Autodesk Fusion 360 part; units mm, degrees
(part 8 of 20)
  spline S469 degree 3 poles (28.0099, -86.4526) (27.9329, -86.3989) (27.7756, -86.2891) (27.5841, -86.2754) (27.4864, -86.2684) knots 0 0 0 0 0.027619 0.056426 0.056426 0.056426 0.056426
  spline S470 degree 3 poles (27.4864, -86.2684) (27.3397, -86.2815) (27.0506, -86.3072) (26.8376, -86.504) (26.7326, -86.6009) knots 0 0 0 0 0.04285 0.084486 0.084486 0.084486 0.084486
  spline S471 degree 3 poles (26.7326, -86.6009) (26.6484, -86.7405) (26.4545, -87.062) (26.447, -87.4395) (26.4427, -87.6531) knots 0 0 0 0 0.048123 0.11083 0.11083 0.11083 0.11083
  spline S472 degree 3 poles (26.4427, -87.6531) (26.4463, -87.8689) (26.4526, -88.2476) (26.6412, -88.5736) (26.7224, -88.7138) knots 0 0 0 0 0.063398 0.111295 0.111295 0.111295 0.111295
  spline S473 degree 3 poles (26.7224, -88.7138) (26.8235, -88.8103) (27.0281, -89.0055) (27.3098, -89.0315) (27.4523, -89.0447) knots 0 0 0 0 0.040675 0.082263 0.082263 0.082263 0.082263
  spline S474 degree 3 poles (27.4523, -89.0447) (27.5666, -89.0365) (27.7895, -89.0205) (27.9687, -88.8876) (28.0559, -88.823) knots 0 0 0 0 0.033628 0.065508 0.065508 0.065508 0.065508
  spline S475 degree 3 poles (28.0559, -88.823) (28.13, -88.733) (28.2935, -88.5344) (28.3383, -88.28) (28.3629, -88.1409) knots 0 0 0 0 0.034396 0.07593 0.07593 0.07593 0.07593
  spline S476 degree 3 poles (21.9679, -37.0341) (21.9715, -36.7658) (21.9781, -36.2826) (22.0973, -35.8148) (22.1504, -35.6068) knots 0 0 0 0 0.080152 0.144341 0.144341 0.144341 0.144341
  spline S477 degree 3 poles (22.1504, -35.6068) (22.215, -35.4399) (22.3376, -35.1234) (22.5787, -34.8854) (22.6927, -34.7729) knots 0 0 0 0 0.052977 0.10048 0.10048 0.10048 0.10048
  spline S478 degree 3 poles (22.6927, -34.7729) (22.8241, -34.6874) (23.0989, -34.5085) (23.427, -34.4895) (23.5982, -34.4795) knots 0 0 0 0 0.046203 0.096661 0.096661 0.096661 0.096661
  spline S479 degree 3 poles (23.5982, -34.4795) (23.726, -34.4851) (23.9715, -34.4958) (24.1964, -34.5943) (24.3042, -34.6415) knots 0 0 0 0 0.037989 0.072993 0.072993 0.072993 0.072993
  spline S480 degree 3 poles (24.3042, -34.6415) (24.4015, -34.7022) (24.5988, -34.8254) (24.736, -35.0134) (24.8056, -35.1088) knots 0 0 0 0 0.034048 0.069103 0.069103 0.069103 0.069103
  spline S481 degree 3 poles (24.8056, -35.1088) (24.8689, -35.2198) (25.0029, -35.4547) (25.0769, -35.715) (25.116, -35.8523) knots 0 0 0 0 0.038176 0.080832 0.080832 0.080832 0.080832
  spline S482 degree 3 poles (25.116, -35.8523) (25.1487, -36.0234) (25.2232, -36.4135) (25.2266, -36.8109) (25.2285, -37.0341) knots 0 0 0 0 0.052146 0.118926 0.118926 0.118926 0.118926
  spline S483 degree 3 poles (25.2285, -37.0341) (25.2249, -37.3007) (25.2183, -37.7815) (25.1003, -38.2472) (25.0477, -38.4546) knots 0 0 0 0 0.079639 0.143634 0.143634 0.143634 0.143634
  spline S484 degree 3 poles (25.0477, -38.4546) (24.9836, -38.6216) (24.8617, -38.9385) (24.621, -39.1773) (24.5072, -39.2903) knots 0 0 0 0 0.052961 0.100531 0.100531 0.100531 0.100531
  spline S485 degree 3 poles (24.5072, -39.2903) (24.3755, -39.3763) (24.0998, -39.5564) (23.7704, -39.5754) (23.5982, -39.5853) knots 0 0 0 0 0.046338 0.097057 0.097057 0.097057 0.097057
  spline S486 degree 3 poles (23.5982, -39.5853) (23.372, -39.566) (22.9307, -39.5283) (22.6159, -39.218) (22.4625, -39.0669) knots 0 0 0 0 0.065835 0.128409 0.128409 0.128409 0.128409
  spline S487 degree 3 poles (22.4625, -39.0669) (22.319, -38.7988) (21.9814, -38.1677) (21.9729, -37.448) (21.9679, -37.0341) knots 0 0 0 0 0.090022 0.211899 0.211899 0.211899 0.211899
  line L97 (28.3868, -38.1733) -> (28.9904, -38.2517)
  spline S488 degree 3 poles (28.9904, -38.2517) (28.9478, -38.4456) (28.866, -38.8173) (28.6076, -39.0957) (28.484, -39.2289) knots 0 0 0 0 0.058356 0.111856 0.111856 0.111856 0.111856
  spline S489 degree 3 poles (28.484, -39.2289) (28.3379, -39.3318) (28.0378, -39.5433) (27.6711, -39.5688) (27.4829, -39.5819) knots 0 0 0 0 0.052559 0.107965 0.107965 0.107965 0.107965
  spline S490 degree 3 poles (27.4829, -39.5819) (27.2499, -39.5644) (26.7983, -39.5304) (26.4541, -39.2376) (26.2875, -39.0958) knots 0 0 0 0 0.068154 0.132052 0.132052 0.132052 0.132052
  spline S491 degree 3 poles (26.2875, -39.0958) (26.156, -38.9051) (25.8681, -38.4877) (25.847, -37.9789) (25.8356, -37.7026) knots 0 0 0 0 0.068157 0.149141 0.149141 0.149141 0.149141
  spline S492 degree 3 poles (25.8356, -37.7026) (25.8419, -37.5174) (25.8539, -37.1649) (25.9733, -36.8333) (26.03, -36.676) knots 0 0 0 0 0.055211 0.105055 0.105055 0.105055 0.105055
  spline S493 degree 3 poles (26.03, -36.676) (26.1022, -36.5391) (26.2444, -36.2695) (26.4973, -36.0996) (26.6218, -36.016) knots 0 0 0 0 0.04564 0.089884 0.089884 0.089884 0.089884
  spline S494 degree 3 poles (26.6218, -36.016) (26.7577, -35.9519) (27.0316, -35.8226) (27.334, -35.8049) (27.4863, -35.7961) knots 0 0 0 0 0.044643 0.089955 0.089955 0.089955 0.089955
  spline S495 degree 3 poles (27.4863, -35.7961) (27.6701, -35.8054) (28.018, -35.8232) (28.3126, -36.0075) (28.4516, -36.0945) knots 0 0 0 0 0.054149 0.102527 0.102527 0.102527 0.102527
  spline S496 degree 3 poles (28.4516, -36.0945) (28.566, -36.208) (28.8051, -36.445) (28.8888, -36.7718) (28.9325, -36.942) knots 0 0 0 0 0.047449 0.099081 0.099081 0.099081 0.099081
  line L98 (28.9325, -36.942) -> (28.3356, -37.0341)
  spline S497 degree 3 poles (28.3356, -37.0341) (28.3047, -36.9227) (28.2473, -36.7153) (28.1013, -36.5579) (28.0338, -36.485) knots 0 0 0 0 0.034086 0.063475 0.063475 0.063475 0.063475
  spline S498 degree 3 poles (28.0338, -36.485) (27.9568, -36.4313) (27.7995, -36.3216) (27.608, -36.3078) (27.5102, -36.3008) knots 0 0 0 0 0.027619 0.056426 0.056426 0.056426 0.056426
  spline S499 degree 3 poles (27.5102, -36.3008) (27.3636, -36.3139) (27.0744, -36.3396) (26.8614, -36.5364) (26.7565, -36.6334) knots 0 0 0 0 0.04285 0.084486 0.084486 0.084486 0.084486
  spline S500 degree 3 poles (26.7565, -36.6334) (26.6723, -36.7729) (26.4784, -37.0944) (26.4708, -37.4719) (26.4666, -37.6855) knots 0 0 0 0 0.048123 0.11083 0.11083 0.11083 0.11083
  spline S501 degree 3 poles (26.4666, -37.6855) (26.4702, -37.9013) (26.4764, -38.28) (26.6651, -38.606) (26.7462, -38.7463) knots 0 0 0 0 0.063398 0.111295 0.111295 0.111295 0.111295
  spline S502 degree 3 poles (26.7462, -38.7463) (26.8474, -38.8427) (27.0519, -39.0379) (27.3337, -39.0639) (27.4761, -39.0771) knots 0 0 0 0 0.040675 0.082263 0.082263 0.082263 0.082263
  spline S503 degree 3 poles (27.4761, -39.0771) (27.5905, -39.0689) (27.8133, -39.0529) (27.9926, -38.92) (28.0798, -38.8554) knots 0 0 0 0 0.033628 0.065508 0.065508 0.065508 0.065508
  spline S504 degree 3 poles (28.0798, -38.8554) (28.1538, -38.7654) (28.3173, -38.5668) (28.3622, -38.3124) (28.3868, -38.1733) knots 0 0 0 0 0.034395 0.07593 0.07593 0.07593 0.07593
  line L99 (29.5157, -39.5) -> (29.5157, -35.8779)
  line L100 (29.5157, -35.8779) -> (30.0648, -35.8779)
  line L101 (30.0648, -35.8779) -> (30.0648, -36.3861)
  spline S505 degree 3 poles (30.0648, -36.3861) (30.1267, -36.3015) (30.2516, -36.131) (30.429, -36.016) (30.5184, -35.9581) knots 0 0 0 0 0.031158 0.062835 0.062835 0.062835 0.062835
  spline S506 degree 3 poles (30.5184, -35.9581) (30.6176, -35.9108) (30.8215, -35.8137) (31.0471, -35.802) (31.163, -35.7961) knots 0 0 0 0 0.032617 0.067048 0.067048 0.067048 0.067048
  spline S507 degree 3 poles (31.163, -35.7961) (31.2875, -35.8008) (31.5199, -35.8096) (31.7269, -35.9145) (31.823, -35.9632) knots 0 0 0 0 0.036859 0.068796 0.068796 0.068796 0.068796
  spline S508 degree 3 poles (31.823, -35.9632) (31.9027, -36.0249) (32.0636, -36.1496) (32.1451, -36.3362) (32.1862, -36.4304) knots 0 0 0 0 0.029725 0.060035 0.060035 0.060035 0.060035
  spline S509 degree 3 poles (32.1862, -36.4304) (32.3364, -36.2455) (32.6275, -35.8869) (33.0839, -35.8257) (33.3049, -35.7961) knots 0 0 0 0 0.068625 0.133023 0.133023 0.133023 0.133023
  spline S510 degree 3 poles (33.3049, -35.7961) (33.47, -35.8045) (33.7779, -35.8202) (34.021, -36.0076) (34.1337, -36.0945) knots 0 0 0 0 0.048244 0.08997 0.08997 0.08997 0.08997
  spline S511 degree 3 poles (34.1337, -36.0945) (34.218, -36.2168) (34.4074, -36.4917) (34.4178, -36.8274) (34.4236, -37.0137) knots 0 0 0 0 0.043695 0.098195 0.098195 0.098195 0.098195
  line L102 (34.4236, -37.0137) -> (34.4236, -39.5)
  line L103 (34.4236, -39.5) -> (33.8131, -39.5)
  line L104 (33.8131, -39.5) -> (33.8131, -37.2183)
  spline S512 degree 3 poles (33.8131, -37.2183) (33.8131, -37.1121) (33.813, -36.9328) (33.7707, -36.7588) (33.7534, -36.6879) knots 0 0 0 0 0.031711 0.053535 0.053535 0.053535 0.053535
  spline S513 degree 3 poles (33.7534, -36.6879) (33.729, -36.6363) (33.6791, -36.5309) (33.5849, -36.4621) (33.5368, -36.427) knots 0 0 0 0 0.016863 0.034394 0.034394 0.034394 0.034394
  spline S514 degree 3 poles (33.5368, -36.427) (33.4811, -36.3982) (33.3657, -36.3384) (33.2357, -36.3316) (33.1685, -36.3281) knots 0 0 0 0 0.018597 0.038532 0.038532 0.038532 0.038532
  spline S515 degree 3 poles (33.1685, -36.3281) (33.0473, -36.3379) (32.8094, -36.3572) (32.6247, -36.5081) (32.5341, -36.5822) knots 0 0 0 0 0.035532 0.069798 0.069798 0.069798 0.069798
  spline S516 degree 3 poles (32.5341, -36.5822) (32.4608, -36.6889) (32.2936, -36.9321) (32.286, -37.229) (32.2817, -37.3956) knots 0 0 0 0 0.038079 0.086792 0.086792 0.086792 0.086792
  line L105 (32.2817, -37.3956) -> (32.2817, -39.5)
  line L106 (32.2817, -39.5) -> (31.6678, -39.5)
  line L107 (31.6678, -39.5) -> (31.6678, -37.1467)
  spline S517 degree 3 poles (31.6678, -37.1467) (31.6654, -37.0246) (31.6611, -36.8078) (31.5613, -36.6164) (31.5177, -36.5328) knots 0 0 0 0 0.036008 0.063954 0.063954 0.063954 0.063954
  spline S518 degree 3 poles (31.5177, -36.5328) (31.4555, -36.4732) (31.3193, -36.3428) (31.1296, -36.3333) (31.0266, -36.3281) knots 0 0 0 0 0.025037 0.054812 0.054812 0.054812 0.054812
  spline S519 degree 3 poles (31.0266, -36.3281) (30.9418, -36.3338) (30.7724, -36.3451) (30.6224, -36.4248) (30.5474, -36.4645) knots 0 0 0 0 0.025172 0.050327 0.050327 0.050327 0.050327
  spline S520 degree 3 poles (30.5474, -36.4645) (30.4788, -36.5162) (30.3385, -36.6218) (30.2657, -36.7818) (30.2285, -36.8636) knots 0 0 0 0 0.025339 0.051812 0.051812 0.051812 0.051812
  spline S521 degree 3 poles (30.2285, -36.8636) (30.1998, -36.9699) (30.133, -37.2174) (30.1308, -37.4742) (30.1296, -37.6207) knots 0 0 0 0 0.032907 0.076633 0.076633 0.076633 0.076633
  line L108 (30.1296, -37.6207) -> (30.1296, -39.5)
  line L109 (30.1296, -39.5) -> (29.5157, -39.5)
  spline S522 degree 3 poles (19.028, -36.7885) (18.9112, -36.7401) (18.6922, -36.6493) (18.5352, -36.4722) (18.4618, -36.3895) knots 0 0 0 0 0.037333 0.070073 0.070073 0.070073 0.070073
  spline S523 degree 3 poles (18.4618, -36.3895) (18.4081, -36.2969) (18.2969, -36.1051) (18.2842, -35.8834) (18.2776, -35.7688) knots 0 0 0 0 0.031652 0.065561 0.065561 0.065561 0.065561
  spline S524 degree 3 poles (18.2776, -35.7688) (18.2938, -35.5943) (18.326, -35.2463) (18.5554, -34.9827) (18.6698, -34.8513) knots 0 0 0 0 0.05117 0.102058 0.102058 0.102058 0.102058
  spline S525 degree 3 poles (18.6698, -34.8513) (18.8165, -34.7429) (19.1259, -34.5144) (19.511, -34.4915) (19.7135, -34.4795) knots 0 0 0 0 0.053536 0.112931 0.112931 0.112931 0.112931
  spline S526 degree 3 poles (19.7135, -34.4795) (19.9176, -34.4921) (20.307, -34.5161) (20.6189, -34.749) (20.7674, -34.8598) knots 0 0 0 0 0.059849 0.114229 0.114229 0.114229 0.114229
  spline S527 degree 3 poles (20.7674, -34.8598) (20.8838, -34.9932) (21.1159, -35.2592) (21.1496, -35.6106) (21.1664, -35.7858) knots 0 0 0 0 0.051706 0.103118 0.103118 0.103118 0.103118
  spline S528 degree 3 poles (21.1664, -35.7858) (21.1597, -35.8968) (21.1464, -36.1132) (21.0372, -36.3002) (20.984, -36.3912) knots 0 0 0 0 0.032847 0.064022 0.064022 0.064022 0.064022
  spline S529 degree 3 poles (20.984, -36.3912) (20.9118, -36.4734) (20.7582, -36.6484) (20.5436, -36.74) (20.4297, -36.7885) knots 0 0 0 0 0.032377 0.06897 0.06897 0.06897 0.06897
  spline S530 degree 3 poles (20.4297, -36.7885) (20.5721, -36.8436) (20.8449, -36.9492) (21.0382, -37.1681) (21.1306, -37.2729) knots 0 0 0 0 0.045038 0.086311 0.086311 0.086311 0.086311
  spline S531 degree 3 poles (21.1306, -37.2729) (21.2007, -37.392) (21.3456, -37.6382) (21.3624, -37.9236) (21.3711, -38.0709) knots 0 0 0 0 0.040859 0.084421 0.084421 0.084421 0.084421
  spline S532 degree 3 poles (21.3711, -38.0709) (21.3526, -38.2758) (21.3157, -38.6833) (21.0498, -38.9941) (20.9175, -39.1487) knots 0 0 0 0 0.060084 0.11955 0.11955 0.11955 0.11955
  spline S533 degree 3 poles (20.9175, -39.1487) (20.7492, -39.276) (20.3968, -39.5425) (19.9547, -39.5706) (19.7237, -39.5853) knots 0 0 0 0 0.061894 0.129627 0.129627 0.129627 0.129627
  spline S534 degree 3 poles (19.7237, -39.5853) (19.4927, -39.5705) (19.0503, -39.5422) (18.6982, -39.2748) (18.53, -39.147) knots 0 0 0 0 0.067741 0.129702 0.129702 0.129702 0.129702
  spline S535 degree 3 poles (18.53, -39.147) (18.3977, -38.9908) (18.1303, -38.6749) (18.0945, -38.2624) (18.0764, -38.0539) knots 0 0 0 0 0.059851 0.120982 0.120982 0.120982 0.120982
  spline S536 degree 3 poles (18.0764, -38.0539) (18.0847, -37.9007) (18.1005, -37.6077) (18.2516, -37.3568) (18.3237, -37.237) knots 0 0 0 0 0.045232 0.08651 0.08651 0.08651 0.08651
  spline S537 degree 3 poles (18.3237, -37.237) (18.4175, -37.1354) (18.6124, -36.9242) (18.886, -36.8349) (19.028, -36.7885) knots 0 0 0 0 0.04079 0.084746 0.084746 0.084746 0.084746
  line L110 (29.4918, -89.4676) -> (29.4918, -85.8455)
  line L111 (29.4918, -85.8455) -> (30.0409, -85.8455)
  line L112 (30.0409, -85.8455) -> (30.0409, -86.3537)
  spline S538 degree 3 poles (30.0409, -86.3537) (30.1029, -86.2691) (30.2277, -86.0986) (30.4051, -85.9836) (30.4945, -85.9256) knots 0 0 0 0 0.031158 0.062835 0.062835 0.062835 0.062835
  spline S539 degree 3 poles (30.4945, -85.9256) (30.5937, -85.8784) (30.7976, -85.7813) (31.0233, -85.7696) (31.1392, -85.7636) knots 0 0 0 0 0.032617 0.067048 0.067048 0.067048 0.067048
  spline S540 degree 3 poles (31.1392, -85.7636) (31.2637, -85.7684) (31.496, -85.7772) (31.703, -85.8821) (31.7991, -85.9308) knots 0 0 0 0 0.036859 0.068796 0.068796 0.068796 0.068796
  spline S541 degree 3 poles (31.7991, -85.9308) (31.8788, -85.9925) (32.0397, -86.1172) (32.1212, -86.3038) (32.1624, -86.398) knots 0 0 0 0 0.029725 0.060035 0.060035 0.060035 0.060035
  spline S542 degree 3 poles (32.1624, -86.398) (32.3125, -86.213) (32.6036, -85.8545) (33.0601, -85.7933) (33.281, -85.7636) knots 0 0 0 0 0.068625 0.133023 0.133023 0.133023 0.133023
  spline S543 degree 3 poles (33.281, -85.7636) (33.4461, -85.772) (33.754, -85.7877) (33.9971, -85.9751) (34.1098, -86.0621) knots 0 0 0 0 0.048244 0.08997 0.08997 0.08997 0.08997
  spline S544 degree 3 poles (34.1098, -86.0621) (34.1941, -86.1844) (34.3835, -86.4593) (34.394, -86.7949) (34.3997, -86.9812) knots 0 0 0 0 0.043695 0.098195 0.098195 0.098195 0.098195
  line L113 (34.3997, -86.9812) -> (34.3997, -89.4676)
  line L114 (34.3997, -89.4676) -> (33.7892, -89.4676)
  line L115 (33.7892, -89.4676) -> (33.7892, -87.1859)
  spline S545 degree 3 poles (33.7892, -87.1859) (33.7892, -87.0797) (33.7892, -86.9003) (33.7468, -86.7264) (33.7295, -86.6555) knots 0 0 0 0 0.031711 0.053535 0.053535 0.053535 0.053535
  spline S546 degree 3 poles (33.7295, -86.6555) (33.7051, -86.6038) (33.6553, -86.4984) (33.561, -86.4297) (33.513, -86.3946) knots 0 0 0 0 0.016863 0.034394 0.034394 0.034394 0.034394
  spline S547 degree 3 poles (33.513, -86.3946) (33.4572, -86.3658) (33.3418, -86.306) (33.2118, -86.2992) (33.1446, -86.2957) knots 0 0 0 0 0.018597 0.038532 0.038532 0.038532 0.038532
  spline S548 degree 3 poles (33.1446, -86.2957) (33.0235, -86.3055) (32.7855, -86.3247) (32.6009, -86.4757) (32.5102, -86.5498) knots 0 0 0 0 0.035532 0.069798 0.069798 0.069798 0.069798
  spline S549 degree 3 poles (32.5102, -86.5498) (32.4369, -86.6565) (32.2698, -86.8996) (32.2621, -87.1966) (32.2578, -87.3632) knots 0 0 0 0 0.038079 0.086792 0.086792 0.086792 0.086792
  line L116 (32.2578, -87.3632) -> (32.2579, -89.4676)
  line L117 (32.2579, -89.4676) -> (31.6439, -89.4676)
  line L118 (31.6439, -89.4676) -> (31.6439, -87.1142)
  spline S550 degree 3 poles (31.6439, -87.1142) (31.6415, -86.9922) (31.6372, -86.7754) (31.5375, -86.584) (31.4939, -86.5003) knots 0 0 0 0 0.036008 0.063954 0.063954 0.063954 0.063954
  spline S551 degree 3 poles (31.4939, -86.5003) (31.4316, -86.4408) (31.2954, -86.3104) (31.1058, -86.3009) (31.0027, -86.2957) knots 0 0 0 0 0.025037 0.054812 0.054812 0.054812 0.054812
  spline S552 degree 3 poles (31.0027, -86.2957) (30.918, -86.3014) (30.7485, -86.3127) (30.5985, -86.3923) (30.5235, -86.4321) knots 0 0 0 0 0.025172 0.050327 0.050327 0.050327 0.050327
  spline S553 degree 3 poles (30.5235, -86.4321) (30.4549, -86.4838) (30.3146, -86.5894) (30.2418, -86.7494) (30.2046, -86.8312) knots 0 0 0 0 0.025339 0.051812 0.051812 0.051812 0.051812
  spline S554 degree 3 poles (30.2046, -86.8312) (30.1759, -86.9375) (30.1091, -87.185) (30.107, -87.4418) (30.1057, -87.5883) knots 0 0 0 0 0.032907 0.076633 0.076633 0.076633 0.076633
  line L119 (30.1057, -87.5883) -> (30.1057, -89.4676)
  line L120 (30.1057, -89.4676) -> (29.4918, -89.4676)
  line L121 (18.1003, -85.1224) -> (18.1003, -84.5324)
  line L122 (18.1003, -84.5324) -> (21.337, -84.5324)
  line L123 (21.337, -84.5324) -> (21.337, -85.0099)
  spline S555 degree 3 poles (21.337, -85.0099) (21.1728, -85.2031) (20.8154, -85.6236) (20.5396, -86.1019) (20.3905, -86.3605) knots 0 0 0 0 0.075903 0.165223 0.165223 0.165223 0.165223
  spline S556 degree 3 poles (20.3905, -86.3605) (20.2435, -86.6418) (19.9525, -87.1986) (19.7607, -87.797) (19.6658, -88.0931) knots 0 0 0 0 0.095012 0.188116 0.188116 0.188116 0.188116
  spline S557 degree 3 poles (19.6658, -88.0931) (19.6097, -88.3112) (19.4935, -88.7629) (19.4519, -89.2274) (19.4304, -89.4676) knots 0 0 0 0 0.06745 0.139654 0.139654 0.139654 0.139654
  line L124 (19.4304, -89.4676) -> (18.7995, -89.4676)
  spline S558 degree 3 poles (18.7995, -89.4676) (18.8147, -89.2495) (18.8485, -88.7675) (18.9667, -88.2987) (19.0314, -88.0419) knots 0 0 0 0 0.065448 0.144689 0.144689 0.144689 0.144689
  spline S559 degree 3 poles (19.0314, -88.0419) (19.1136, -87.7653) (19.2788, -87.2097) (19.5375, -86.6909) (19.6675, -86.4304) knots 0 0 0 0 0.086392 0.173544 0.173544 0.173544 0.173544
  spline S560 degree 3 poles (19.6675, -86.4304) (19.8031, -86.1874) (20.0603, -85.7265) (20.3922, -85.3163) (20.5491, -85.1224) knots 0 0 0 0 0.083307 0.157996 0.157996 0.157996 0.157996
  line L125 (20.5491, -85.1224) -> (18.1003, -85.1224)
  line L126 (29.4918, -139.5) -> (29.4918, -135.8779)
  line L127 (29.4918, -135.8779) -> (30.0409, -135.8779)
  line L128 (30.0409, -135.8779) -> (30.0409, -136.3861)
  spline S561 degree 3 poles (30.0409, -136.3861) (30.1028, -136.3015) (30.2277, -136.131) (30.4051, -136.016) (30.4945, -135.9581) knots 0 0 0 0 0.031158 0.062835 0.062835 0.062835 0.062835
  spline S562 degree 3 poles (30.4945, -135.9581) (30.5937, -135.9108) (30.7976, -135.8137) (31.0232, -135.802) (31.1391, -135.7961) knots 0 0 0 0 0.032617 0.067048 0.067048 0.067048 0.067048
  spline S563 degree 3 poles (31.1391, -135.7961) (31.2636, -135.8008) (31.496, -135.8096) (31.703, -135.9145) (31.7991, -135.9632) knots 0 0 0 0 0.036859 0.068796 0.068796 0.068796 0.068796
  spline S564 degree 3 poles (31.7991, -135.9632) (31.8788, -136.0249) (32.0397, -136.1496) (32.1212, -136.3362) (32.1623, -136.4304) knots 0 0 0 0 0.029725 0.060035 0.060035 0.060035 0.060035
  spline S565 degree 3 poles (32.1623, -136.4304) (32.3125, -136.2455) (32.6036, -135.8869) (33.0601, -135.8257) (33.281, -135.7961) knots 0 0 0 0 0.068625 0.133023 0.133023 0.133023 0.133023
  spline S566 degree 3 poles (33.281, -135.7961) (33.4461, -135.8045) (33.754, -135.8201) (33.9971, -136.0076) (34.1098, -136.0945) knots 0 0 0 0 0.048244 0.08997 0.08997 0.08997 0.08997
  spline S567 degree 3 poles (34.1098, -136.0945) (34.1941, -136.2168) (34.3835, -136.4917) (34.3939, -136.8274) (34.3997, -137.0137) knots 0 0 0 0 0.043695 0.098195 0.098195 0.098195 0.098195
  line L129 (34.3997, -137.0137) -> (34.3997, -139.5)
  line L130 (34.3997, -139.5) -> (33.7892, -139.5)
  line L131 (33.7892, -139.5) -> (33.7892, -137.2183)
  spline S568 degree 3 poles (33.7892, -137.2183) (33.7892, -137.1121) (33.7891, -136.9328) (33.7468, -136.7588) (33.7295, -136.6879) knots 0 0 0 0 0.031711 0.053535 0.053535 0.053535 0.053535
  spline S569 degree 3 poles (33.7295, -136.6879) (33.7051, -136.6363) (33.6552, -136.5309) (33.561, -136.4621) (33.5129, -136.427) knots 0 0 0 0 0.016863 0.034394 0.034394 0.034394 0.034394
  spline S570 degree 3 poles (33.5129, -136.427) (33.4572, -136.3982) (33.3418, -136.3384) (33.2118, -136.3316) (33.1446, -136.3281) knots 0 0 0 0 0.018597 0.038532 0.038532 0.038532 0.038532
  spline S571 degree 3 poles (33.1446, -136.3281) (33.0235, -136.3379) (32.7855, -136.3572) (32.6009, -136.5081) (32.5102, -136.5822) knots 0 0 0 0 0.035532 0.069798 0.069798 0.069798 0.069798
  spline S572 degree 3 poles (32.5102, -136.5822) (32.4369, -136.6889) (32.2697, -136.9321) (32.2621, -137.229) (32.2578, -137.3956) knots 0 0 0 0 0.038079 0.086792 0.086792 0.086792 0.086792
  line L132 (32.2578, -137.3956) -> (32.2578, -139.5)
  line L133 (32.2578, -139.5) -> (31.6439, -139.5)
  line L134 (31.6439, -139.5) -> (31.6439, -137.1467)
  spline S573 degree 3 poles (31.6439, -137.1467) (31.6415, -137.0246) (31.6372, -136.8078) (31.5374, -136.6164) (31.4938, -136.5328) knots 0 0 0 0 0.036008 0.063954 0.063954 0.063954 0.063954
  spline S574 degree 3 poles (31.4938, -136.5328) (31.4316, -136.4732) (31.2954, -136.3428) (31.1057, -136.3333) (31.0027, -136.3281) knots 0 0 0 0 0.025037 0.054812 0.054812 0.054812 0.054812
  spline S575 degree 3 poles (31.0027, -136.3281) (30.918, -136.3338) (30.7485, -136.3451) (30.5985, -136.4247) (30.5235, -136.4645) knots 0 0 0 0 0.025172 0.050327 0.050327 0.050327 0.050327
  spline S576 degree 3 poles (30.5235, -136.4645) (30.4549, -136.5162) (30.3146, -136.6218) (30.2418, -136.7818) (30.2046, -136.8636) knots 0 0 0 0 0.025339 0.051812 0.051812 0.051812 0.051812
  spline S577 degree 3 poles (30.2046, -136.8636) (30.1759, -136.9699) (30.1091, -137.2174) (30.1069, -137.4742) (30.1057, -137.6207) knots 0 0 0 0 0.032907 0.076633 0.076633 0.076633 0.076633
  line L135 (30.1057, -137.6207) -> (30.1057, -139.5)
  line L136 (30.1057, -139.5) -> (29.4918, -139.5)
  line L137 (18.1003, -135.1548) -> (18.1003, -134.5648)
  line L138 (18.1003, -134.5648) -> (21.337, -134.5648)
  line L139 (21.337, -134.5648) -> (21.337, -135.0423)
  spline S578 degree 3 poles (21.337, -135.0423) (21.1728, -135.2355) (20.8153, -135.656) (20.5396, -136.1343) (20.3905, -136.3929) knots 0 0 0 0 0.075903 0.165223 0.165223 0.165223 0.165223
  spline S579 degree 3 poles (20.3905, -136.3929) (20.2435, -136.6742) (19.9525, -137.2311) (19.7607, -137.8294) (19.6657, -138.1255) knots 0 0 0 0 0.095012 0.188116 0.188116 0.188116 0.188116
  spline S580 degree 3 poles (19.6657, -138.1255) (19.6096, -138.3436) (19.4935, -138.7953) (19.4519, -139.2598) (19.4304, -139.5) knots 0 0 0 0 0.06745 0.139654 0.139654 0.139654 0.139654
  line L140 (19.4304, -139.5) -> (18.7994, -139.5)
  spline S581 degree 3 poles (18.7994, -139.5) (18.8147, -139.282) (18.8485, -138.7999) (18.9666, -138.3311) (19.0314, -138.0744) knots 0 0 0 0 0.065448 0.144689 0.144689 0.144689 0.144689
  spline S582 degree 3 poles (19.0314, -138.0744) (19.1136, -137.7977) (19.2788, -137.2421) (19.5375, -136.7233) (19.6674, -136.4628) knots 0 0 0 0 0.086392 0.173544 0.173544 0.173544 0.173544
  spline S583 degree 3 poles (19.6674, -136.4628) (19.8031, -136.2198) (20.0602, -135.7589) (20.3922, -135.3487) (20.5491, -135.1548) knots 0 0 0 0 0.083307 0.157996 0.157996 0.157996 0.157996
  line L141 (20.5491, -135.1548) -> (18.1003, -135.1548)
  line L142 (29.5259, -189.5) -> (29.5259, -185.8779)
  line L143 (29.5259, -185.8779) -> (30.075, -185.8779)
  line L144 (30.075, -185.8779) -> (30.075, -186.3861)
  spline S584 degree 3 poles (30.075, -186.3861) (30.137, -186.3015) (30.2618, -186.131) (30.4392, -186.016) (30.5287, -185.958) knots 0 0 0 0 0.031158 0.062835 0.062835 0.062835 0.062835
  spline S585 degree 3 poles (30.5287, -185.958) (30.6278, -185.9108) (30.8317, -185.8137) (31.0574, -185.802) (31.1733, -185.796) knots 0 0 0 0 0.032617 0.067048 0.067048 0.067048 0.067048
  spline S586 degree 3 poles (31.1733, -185.796) (31.2978, -185.8008) (31.5301, -185.8096) (31.7371, -185.9145) (31.8332, -185.9632) knots 0 0 0 0 0.036859 0.068796 0.068796 0.068796 0.068796
  spline S587 degree 3 poles (31.8332, -185.9632) (31.9129, -186.0249) (32.0738, -186.1496) (32.1553, -186.3362) (32.1965, -186.4304) knots 0 0 0 0 0.029725 0.060035 0.060035 0.060035 0.060035
  spline S588 degree 3 poles (32.1965, -186.4304) (32.3466, -186.2454) (32.6378, -185.8869) (33.0942, -185.8257) (33.3151, -185.796) knots 0 0 0 0 0.068625 0.133023 0.133023 0.133023 0.133023
  spline S589 degree 3 poles (33.3151, -185.796) (33.4802, -185.8045) (33.7881, -185.8201) (34.0312, -186.0076) (34.1439, -186.0945) knots 0 0 0 0 0.048244 0.08997 0.08997 0.08997 0.08997
  spline S590 degree 3 poles (34.1439, -186.0945) (34.2282, -186.2168) (34.4177, -186.4917) (34.4281, -186.8273) (34.4338, -187.0136) knots 0 0 0 0 0.043695 0.098195 0.098195 0.098195 0.098195
  line L145 (34.4338, -187.0136) -> (34.4338, -189.5)
  line L146 (34.4338, -189.5) -> (33.8233, -189.5)
  line L147 (33.8233, -189.5) -> (33.8233, -187.2183)
  spline S591 degree 3 poles (33.8233, -187.2183) (33.8233, -187.1121) (33.8233, -186.9327) (33.7809, -186.7588) (33.7636, -186.6879) knots 0 0 0 0 0.031711 0.053535 0.053535 0.053535 0.053535
  spline S592 degree 3 poles (33.7636, -186.6879) (33.7392, -186.6362) (33.6894, -186.5308) (33.5951, -186.4621) (33.5471, -186.427) knots 0 0 0 0 0.016863 0.034394 0.034394 0.034394 0.034394
  spline S593 degree 3 poles (33.5471, -186.427) (33.4914, -186.3982) (33.3759, -186.3384) (33.246, -186.3316) (33.1787, -186.3281) knots 0 0 0 0 0.018597 0.038532 0.038532 0.038532 0.038532
  spline S594 degree 3 poles (33.1787, -186.3281) (33.0576, -186.3379) (32.8196, -186.3571) (32.635, -186.5081) (32.5443, -186.5822) knots 0 0 0 0 0.035532 0.069798 0.069798 0.069798 0.069798
  spline S595 degree 3 poles (32.5443, -186.5822) (32.471, -186.6889) (32.3039, -186.932) (32.2962, -187.229) (32.292, -187.3956) knots 0 0 0 0 0.038079 0.086792 0.086792 0.086792 0.086792
  line L148 (32.292, -187.3956) -> (32.292, -189.5)
  line L149 (32.292, -189.5) -> (31.678, -189.5)
  line L150 (31.678, -189.5) -> (31.678, -187.1467)
  spline S596 degree 3 poles (31.678, -187.1467) (31.6756, -187.0246) (31.6713, -186.8078) (31.5716, -186.6164) (31.528, -186.5327) knots 0 0 0 0 0.036008 0.063954 0.063954 0.063954 0.063954
  spline S597 degree 3 poles (31.528, -186.5327) (31.4658, -186.4732) (31.3295, -186.3428) (31.1399, -186.3333) (31.0368, -186.3281) knots 0 0 0 0 0.025037 0.054812 0.054812 0.054812 0.054812
  spline S598 degree 3 poles (31.0368, -186.3281) (30.9521, -186.3338) (30.7826, -186.3451) (30.6326, -186.4247) (30.5576, -186.4645) knots 0 0 0 0 0.025172 0.050327 0.050327 0.050327 0.050327
  spline S599 degree 3 poles (30.5576, -186.4645) (30.489, -186.5162) (30.3487, -186.6218) (30.2759, -186.7818) (30.2388, -186.8636) knots 0 0 0 0 0.025339 0.051812 0.051812 0.051812 0.051812
  spline S600 degree 3 poles (30.2388, -186.8636) (30.21, -186.9699) (30.1432, -187.2174) (30.1411, -187.4742) (30.1398, -187.6207) knots 0 0 0 0 0.032907 0.076633 0.076633 0.076633 0.076633
  line L151 (30.1398, -187.6207) -> (30.1398, -189.5)
  line L152 (30.1398, -189.5) -> (29.5259, -189.5)
  line L153 (21.279, -185.7244) -> (20.6685, -185.7722)
  spline S601 degree 3 poles (20.6685, -185.7722) (20.6425, -185.6649) (20.5967, -185.4753) (20.485, -185.3161) (20.4366, -185.2469) knots 0 0 0 0 0.032737 0.057863 0.057863 0.057863 0.057863
  spline S602 degree 3 poles (20.4366, -185.2469) (20.3486, -185.1703) (20.1722, -185.0168) (19.9394, -184.9952) (19.8227, -184.9843) knots 0 0 0 0 0.034068 0.068298 0.068298 0.068298 0.068298
  spline S603 degree 3 poles (19.8227, -184.9843) (19.7285, -184.9907) (19.5433, -185.0032) (19.3853, -185.1003) (19.3076, -185.148) knots 0 0 0 0 0.027843 0.054766 0.054766 0.054766 0.054766
  spline S604 degree 3 poles (19.3076, -185.148) (19.2148, -185.2299) (19.0188, -185.4028) (18.9086, -185.6403) (18.8506, -185.7654) knots 0 0 0 0 0.036718 0.077555 0.077555 0.077555 0.077555
  spline S605 degree 3 poles (18.8506, -185.7654) (18.8017, -185.9283) (18.6886, -186.3047) (18.681, -186.6983) (18.6767, -186.9216) knots 0 0 0 0 0.050812 0.1174 0.1174 0.1174 0.1174
  spline S606 degree 3 poles (18.6767, -186.9216) (18.753, -186.8171) (18.9011, -186.6144) (19.1152, -186.4836) (19.219, -186.4202) knots 0 0 0 0 0.038374 0.074495 0.074495 0.074495 0.074495
  spline S607 degree 3 poles (19.219, -186.4202) (19.3267, -186.3724) (19.5409, -186.2776) (19.7747, -186.2635) (19.8909, -186.2565) knots 0 0 0 0 0.035048 0.069654 0.069654 0.069654 0.069654
  spline S608 degree 3 poles (19.8909, -186.2565) (20.0883, -186.2757) (20.485, -186.3143) (20.7853, -186.5766) (20.9362, -186.7084) knots 0 0 0 0 0.057942 0.116462 0.116462 0.116462 0.116462
  spline S609 degree 3 poles (20.9362, -186.7084) (21.062, -186.8743) (21.3235, -187.2192) (21.3526, -187.6519) (21.3677, -187.8765) knots 0 0 0 0 0.061076 0.12698 0.12698 0.12698 0.12698
  spline S610 degree 3 poles (21.3677, -187.8765) (21.3596, -188.0299) (21.3435, -188.3336) (21.2239, -188.6131) (21.1647, -188.7514) knots 0 0 0 0 0.045687 0.090433 0.090433 0.090433 0.090433
  spline S611 degree 3 poles (21.1647, -188.7514) (21.0922, -188.8773) (20.9503, -189.1236) (20.7197, -189.2894) (20.6071, -189.3704) knots 0 0 0 0 0.043053 0.084173 0.084173 0.084173 0.084173
  spline S612 degree 3 poles (20.6071, -189.3704) (20.4833, -189.4331) (20.2303, -189.5612) (19.9469, -189.5771) (19.8022, -189.5853) knots 0 0 0 0 0.041145 0.084115 0.084115 0.084115 0.084115
  spline S613 degree 3 poles (19.8022, -189.5853) (19.5589, -189.5626) (19.0767, -189.5177) (18.7248, -189.1854) (18.5505, -189.0208) knots 0 0 0 0 0.071077 0.140887 0.140887 0.140887 0.140887
  spline S614 degree 3 poles (18.5505, -189.0208) (18.41, -188.7773) (18.0802, -188.2056) (18.0713, -187.5415) (18.0662, -187.1603) knots 0 0 0 0 0.083095 0.195067 0.195067 0.195067 0.195067
  spline S615 degree 3 poles (18.0662, -187.1603) (18.0727, -186.7324) (18.084, -185.9831) (18.4463, -185.3319) (18.6016, -185.0525) knots 0 0 0 0 0.125884 0.220443 0.220443 0.220443 0.220443
  spline S616 degree 3 poles (18.6016, -185.0525) (18.7734, -184.8854) (19.1238, -184.5445) (19.6115, -184.5015) (19.8602, -184.4795) knots 0 0 0 0 0.069661 0.142118 0.142118 0.142118 0.142118
  spline S617 degree 3 poles (19.8602, -184.4795) (20.0449, -184.4907) (20.3984, -184.512) (20.6885, -184.7139) (20.8271, -184.8104) knots 0 0 0 0 0.054308 0.103968 0.103968 0.103968 0.103968
  spline S618 degree 3 poles (20.8271, -184.8104) (20.9406, -184.9351) (21.178, -185.196) (21.2444, -185.5432) (21.279, -185.7244) knots 0 0 0 0 0.049602 0.103747 0.103747 0.103747 0.103747
  line L154 (29.5256, -239.5001) -> (29.5256, -235.878)
  line L155 (29.5256, -235.878) -> (30.0747, -235.878)
  line L156 (30.0747, -235.878) -> (30.0747, -236.3862)
  spline S619 degree 3 poles (30.0747, -236.3862) (30.1366, -236.3016) (30.2615, -236.1311) (30.4389, -236.0161) (30.5283, -235.9582) knots 0 0 0 0 0.031158 0.062835 0.062835 0.062835 0.062835
  spline S620 degree 3 poles (30.5283, -235.9582) (30.6275, -235.9109) (30.8314, -235.8138) (31.0571, -235.8022) (31.173, -235.7962) knots 0 0 0 0 0.032617 0.067048 0.067048 0.067048 0.067048
  spline S621 degree 3 poles (31.173, -235.7962) (31.2975, -235.8009) (31.5298, -235.8098) (31.7368, -235.9146) (31.8329, -235.9633) knots 0 0 0 0 0.036859 0.068796 0.068796 0.068796 0.068796
  spline S622 degree 3 poles (31.8329, -235.9633) (31.9126, -236.025) (32.0735, -236.1497) (32.155, -236.3363) (32.1961, -236.4305) knots 0 0 0 0 0.029725 0.060035 0.060035 0.060035 0.060035
  spline S623 degree 3 poles (32.1961, -236.4305) (32.3463, -236.2456) (32.6374, -235.887) (33.0939, -235.8258) (33.3148, -235.7962) knots 0 0 0 0 0.068625 0.133023 0.133023 0.133023 0.133023
  spline S624 degree 3 poles (33.3148, -235.7962) (33.4799, -235.8046) (33.7878, -235.8203) (34.0309, -236.0077) (34.1436, -236.0946) knots 0 0 0 0 0.048244 0.08997 0.08997 0.08997 0.08997
  spline S625 degree 3 poles (34.1436, -236.0946) (34.2279, -236.2169) (34.4173, -236.4919) (34.4277, -236.8275) (34.4335, -237.0138) knots 0 0 0 0 0.043695 0.098195 0.098195 0.098195 0.098195
  line L157 (34.4335, -237.0138) -> (34.4335, -239.5001)
  line L158 (34.4335, -239.5001) -> (33.823, -239.5001)
  line L159 (33.823, -239.5001) -> (33.823, -237.2184)
  spline S626 degree 3 poles (33.823, -237.2184) (33.823, -237.1122) (33.8229, -236.9329) (33.7806, -236.759) (33.7633, -236.6881) knots 0 0 0 0 0.031711 0.053535 0.053535 0.053535 0.053535
  spline S627 degree 3 poles (33.7633, -236.6881) (33.7389, -236.6364) (33.6891, -236.531) (33.5948, -236.4622) (33.5468, -236.4271) knots 0 0 0 0 0.016863 0.034394 0.034394 0.034394 0.034394
  spline S628 degree 3 poles (33.5468, -236.4271) (33.491, -236.3983) (33.3756, -236.3386) (33.2456, -236.3318) (33.1784, -236.3282) knots 0 0 0 0 0.018597 0.038532 0.038532 0.038532 0.038532
  spline S629 degree 3 poles (33.1784, -236.3282) (33.0573, -236.338) (32.8193, -236.3573) (32.6347, -236.5082) (32.544, -236.5823) knots 0 0 0 0 0.035532 0.069798 0.069798 0.069798 0.069798
  spline S630 degree 3 poles (32.544, -236.5823) (32.4707, -236.689) (32.3035, -236.9322) (32.2959, -237.2291) (32.2916, -237.3958) knots 0 0 0 0 0.038079 0.086792 0.086792 0.086792 0.086792
  line L160 (32.2916, -237.3958) -> (32.2916, -239.5001)
  line L161 (32.2916, -239.5001) -> (31.6777, -239.5001)
  line L162 (31.6777, -239.5001) -> (31.6777, -237.1468)
  spline S631 degree 3 poles (31.6777, -237.1468) (31.6753, -237.0247) (31.671, -236.808) (31.5713, -236.6165) (31.5277, -236.5329) knots 0 0 0 0 0.036008 0.063954 0.063954 0.063954 0.063954
  spline S632 degree 3 poles (31.5277, -236.5329) (31.4654, -236.4733) (31.3292, -236.3429) (31.1396, -236.3334) (31.0365, -236.3282) knots 0 0 0 0 0.025037 0.054812 0.054812 0.054812 0.054812
  spline S633 degree 3 poles (31.0365, -236.3282) (30.9518, -236.3339) (30.7823, -236.3452) (30.6323, -236.4249) (30.5573, -236.4646) knots 0 0 0 0 0.025172 0.050327 0.050327 0.050327 0.050327
  spline S634 degree 3 poles (30.5573, -236.4646) (30.4887, -236.5163) (30.3484, -236.6219) (30.2756, -236.7819) (30.2384, -236.8637) knots 0 0 0 0 0.025339 0.051812 0.051812 0.051812 0.051812
  spline S635 degree 3 poles (30.2384, -236.8637) (30.2097, -236.97) (30.1429, -237.2175) (30.1407, -237.4743) (30.1395, -237.6208) knots 0 0 0 0 0.032907 0.076633 0.076633 0.076633 0.076633
  line L163 (30.1395, -237.6208) -> (30.1395, -239.5001)
  line L164 (30.1395, -239.5001) -> (29.5256, -239.5001)
  line L165 (21.2787, -235.7245) -> (20.6682, -235.7722)
  spline S636 degree 3 poles (20.6682, -235.7722) (20.6422, -235.6649) (20.5964, -235.4754) (20.4847, -235.3161) (20.4363, -235.247) knots 0 0 0 0 0.032737 0.057863 0.057863 0.057863 0.057863
  spline S637 degree 3 poles (20.4363, -235.247) (20.3483, -235.1704) (20.1719, -235.0168) (19.9391, -234.9952) (19.8223, -234.9843) knots 0 0 0 0 0.034068 0.068298 0.068298 0.068298 0.068298
  spline S638 degree 3 poles (19.8223, -234.9843) (19.7282, -234.9907) (19.543, -235.0032) (19.385, -235.1003) (19.3073, -235.148) knots 0 0 0 0 0.027843 0.054766 0.054766 0.054766 0.054766
  spline S639 degree 3 poles (19.3073, -235.148) (19.2145, -235.2299) (19.0185, -235.4028) (18.9083, -235.6403) (18.8503, -235.7654) knots 0 0 0 0 0.036718 0.077555 0.077555 0.077555 0.077555
  spline S640 degree 3 poles (18.8503, -235.7654) (18.8014, -235.9283) (18.6883, -236.3047) (18.6807, -236.6983) (18.6764, -236.9216) knots 0 0 0 0 0.050812 0.1174 0.1174 0.1174 0.1174
  spline S641 degree 3 poles (18.6764, -236.9216) (18.7527, -236.8172) (18.9008, -236.6145) (19.1149, -236.4836) (19.2187, -236.4202) knots 0 0 0 0 0.038374 0.074495 0.074495 0.074495 0.074495
  spline S642 degree 3 poles (19.2187, -236.4202) (19.3264, -236.3725) (19.5406, -236.2776) (19.7744, -236.2635) (19.8906, -236.2565) knots 0 0 0 0 0.035048 0.069654 0.069654 0.069654 0.069654
  spline S643 degree 3 poles (19.8906, -236.2565) (20.0879, -236.2757) (20.4847, -236.3143) (20.785, -236.5766) (20.9359, -236.7084) knots 0 0 0 0 0.057942 0.116462 0.116462 0.116462 0.116462
  spline S644 degree 3 poles (20.9359, -236.7084) (21.0617, -236.8743) (21.3232, -237.2192) (21.3523, -237.652) (21.3673, -237.8766) knots 0 0 0 0 0.061076 0.12698 0.12698 0.12698 0.12698
  spline S645 degree 3 poles (21.3673, -237.8766) (21.3592, -238.03) (21.3432, -238.3336) (21.2236, -238.6131) (21.1644, -238.7514) knots 0 0 0 0 0.045687 0.090433 0.090433 0.090433 0.090433
  spline S646 degree 3 poles (21.1644, -238.7514) (21.0919, -238.8774) (20.95, -239.1236) (20.7194, -239.2894) (20.6068, -239.3704) knots 0 0 0 0 0.043053 0.084173 0.084173 0.084173 0.084173
  spline S647 degree 3 poles (20.6068, -239.3704) (20.483, -239.4331) (20.2299, -239.5612) (19.9466, -239.5771) (19.8018, -239.5853) knots 0 0 0 0 0.041145 0.084115 0.084115 0.084115 0.084115
  spline S648 degree 3 poles (19.8018, -239.5853) (19.5586, -239.5626) (19.0764, -239.5177) (18.7245, -239.1855) (18.5501, -239.0208) knots 0 0 0 0 0.071077 0.140887 0.140887 0.140887 0.140887
  spline S649 degree 3 poles (18.5501, -239.0208) (18.4097, -238.7773) (18.0799, -238.2056) (18.071, -237.5415) (18.0659, -237.1603) knots 0 0 0 0 0.083095 0.195067 0.195067 0.195067 0.195067
  spline S650 degree 3 poles (18.0659, -237.1603) (18.0723, -236.7324) (18.0837, -235.9831) (18.4459, -235.3319) (18.6013, -235.0525) knots 0 0 0 0 0.125884 0.220443 0.220443 0.220443 0.220443
  spline S651 degree 3 poles (18.6013, -235.0525) (18.7731, -234.8854) (19.1235, -234.5445) (19.6112, -234.5015) (19.8599, -234.4796) knots 0 0 0 0 0.069661 0.142118 0.142118 0.142118 0.142118
  spline S652 degree 3 poles (19.8599, -234.4796) (20.0446, -234.4907) (20.3981, -234.5121) (20.6882, -234.714) (20.8268, -234.8104) knots 0 0 0 0 0.054308 0.103968 0.103968 0.103968 0.103968
  spline S653 degree 3 poles (20.8268, -234.8104) (20.9403, -234.9351) (21.1777, -235.196) (21.2441, -235.5432) (21.2787, -235.7245) knots 0 0 0 0 0.049602 0.103747 0.103747 0.103747 0.103747
  line L166 (29.5124, -289.4659) -> (29.5124, -285.8438)
  line L167 (29.5124, -285.8438) -> (30.0615, -285.8438)
  line L168 (30.0615, -285.8438) -> (30.0615, -286.3519)
  spline S654 degree 3 poles (30.0615, -286.3519) (30.1234, -286.2674) (30.2483, -286.0968) (30.4257, -285.9819) (30.5151, -285.9239) knots 0 0 0 0 0.031158 0.062835 0.062835 0.062835 0.062835
  spline S655 degree 3 poles (30.5151, -285.9239) (30.6143, -285.8767) (30.8182, -285.7796) (31.0438, -285.7679) (31.1597, -285.7619) knots 0 0 0 0 0.032617 0.067048 0.067048 0.067048 0.067048
  spline S656 degree 3 poles (31.1597, -285.7619) (31.2842, -285.7666) (31.5166, -285.7755) (31.7236, -285.8803) (31.8197, -285.929) knots 0 0 0 0 0.036859 0.068796 0.068796 0.068796 0.068796
  spline S657 degree 3 poles (31.8197, -285.929) (31.8994, -285.9907) (32.0603, -286.1154) (32.1418, -286.302) (32.1829, -286.3963) knots 0 0 0 0 0.029725 0.060035 0.060035 0.060035 0.060035
  spline S658 degree 3 poles (32.1829, -286.3963) (32.3331, -286.2113) (32.6242, -285.8528) (33.0806, -285.7915) (33.3016, -285.7619) knots 0 0 0 0 0.068625 0.133023 0.133023 0.133023 0.133023
  spline S659 degree 3 poles (33.3016, -285.7619) (33.4667, -285.7703) (33.7746, -285.786) (34.0177, -285.9734) (34.1304, -286.0603) knots 0 0 0 0 0.048244 0.08997 0.08997 0.08997 0.08997
  spline S660 degree 3 poles (34.1304, -286.0603) (34.2147, -286.1826) (34.4041, -286.4576) (34.4145, -286.7932) (34.4203, -286.9795) knots 0 0 0 0 0.043695 0.098195 0.098195 0.098195 0.098195
  line L169 (34.4203, -286.9795) -> (34.4203, -289.4658)
  line L170 (34.4203, -289.4658) -> (33.8098, -289.4658)
  line L171 (33.8098, -289.4658) -> (33.8098, -287.1841)
  spline S661 degree 3 poles (33.8098, -287.1841) (33.8098, -287.0779) (33.8097, -286.8986) (33.7674, -286.7247) (33.7501, -286.6538) knots 0 0 0 0 0.031711 0.053535 0.053535 0.053535 0.053535
  spline S662 degree 3 poles (33.7501, -286.6538) (33.7257, -286.6021) (33.6758, -286.4967) (33.5816, -286.4279) (33.5335, -286.3929) knots 0 0 0 0 0.016863 0.034394 0.034394 0.034394 0.034394
  spline S663 degree 3 poles (33.5335, -286.3929) (33.4778, -286.364) (33.3624, -286.3043) (33.2324, -286.2975) (33.1652, -286.294) knots 0 0 0 0 0.018597 0.038532 0.038532 0.038532 0.038532
  spline S664 degree 3 poles (33.1652, -286.294) (33.044, -286.3038) (32.8061, -286.323) (32.6215, -286.4739) (32.5308, -286.548) knots 0 0 0 0 0.035532 0.069798 0.069798 0.069798 0.069798
  spline S665 degree 3 poles (32.5308, -286.548) (32.4575, -286.6547) (32.2903, -286.8979) (32.2827, -287.1948) (32.2784, -287.3615) knots 0 0 0 0 0.038079 0.086792 0.086792 0.086792 0.086792
  line L172 (32.2784, -287.3615) -> (32.2784, -289.4659)
  line L173 (32.2784, -289.4659) -> (31.6645, -289.4659)
  line L174 (31.6645, -289.4659) -> (31.6645, -287.1125)
  spline S666 degree 3 poles (31.6645, -287.1125) (31.6621, -286.9905) (31.6578, -286.7737) (31.558, -286.5822) (31.5144, -286.4986) knots 0 0 0 0 0.036008 0.063954 0.063954 0.063954 0.063954
  spline S667 degree 3 poles (31.5144, -286.4986) (31.4522, -286.439) (31.316, -286.3086) (31.1263, -286.2991) (31.0233, -286.294) knots 0 0 0 0 0.025037 0.054812 0.054812 0.054812 0.054812
  spline S668 degree 3 poles (31.0233, -286.294) (30.9385, -286.2996) (30.7691, -286.311) (30.6191, -286.3906) (30.5441, -286.4304) knots 0 0 0 0 0.025172 0.050327 0.050327 0.050327 0.050327
  spline S669 degree 3 poles (30.5441, -286.4304) (30.4755, -286.482) (30.3352, -286.5877) (30.2624, -286.7477) (30.2252, -286.8294) knots 0 0 0 0 0.025339 0.051812 0.051812 0.051812 0.051812
  spline S670 degree 3 poles (30.2252, -286.8294) (30.1965, -286.9357) (30.1297, -287.1833) (30.1275, -287.4401) (30.1263, -287.5866) knots 0 0 0 0 0.032907 0.076633 0.076633 0.076633 0.076633
  line L175 (30.1263, -287.5866) -> (30.1263, -289.4659)
  line L176 (30.1263, -289.4659) -> (29.5124, -289.4659)
  line L177 (18.0799, -288.1562) -> (18.7245, -288.1016)
  spline S671 degree 3 poles (18.7245, -288.1016) (18.7522, -288.2449) (18.8035, -288.5098) (18.9773, -288.7151) (19.0571, -288.8093) knots 0 0 0 0 0.042908 0.079365 0.079365 0.079365 0.079365
  spline S672 degree 3 poles (19.0571, -288.8093) (19.1493, -288.8785) (19.3359, -289.0184) (19.5686, -289.037) (19.6863, -289.0464) knots 0 0 0 0 0.033826 0.068485 0.068485 0.068485 0.068485
  spline S673 degree 3 poles (19.6863, -289.0464) (19.8288, -289.0321) (20.1156, -289.0033) (20.3292, -288.8096) (20.4367, -288.7121) knots 0 0 0 0 0.041772 0.0841 0.0841 0.0841 0.0841
  spline S674 degree 3 poles (20.4367, -288.7121) (20.5261, -288.5871) (20.7153, -288.3226) (20.7339, -287.997) (20.7436, -287.8254) knots 0 0 0 0 0.045186 0.095569 0.095569 0.095569 0.095569
  spline S675 degree 3 poles (20.7436, -287.8254) (20.7346, -287.663) (20.7175, -287.3567) (20.5346, -287.1117) (20.4486, -286.9966) knots 0 0 0 0 0.047557 0.089725 0.089725 0.089725 0.089725
  spline S676 degree 3 poles (20.4486, -286.9966) (20.3401, -286.9081) (20.1155, -286.7248) (19.8259, -286.7039) (19.6761, -286.693) knots 0 0 0 0 0.040971 0.08482 0.08482 0.08482 0.08482
  spline S677 degree 3 poles (19.6761, -286.693) (19.5805, -286.6982) (19.3931, -286.7082) (19.2236, -286.7885) (19.1406, -286.8278) knots 0 0 0 0 0.028423 0.055689 0.055689 0.055689 0.055689
  spline S678 degree 3 poles (19.1406, -286.8278) (19.0658, -286.8753) (18.9189, -286.9685) (18.8159, -287.1086) (18.7655, -287.1773) knots 0 0 0 0 0.026342 0.051681 0.051681 0.051681 0.051681
  line L178 (18.7655, -287.1773) -> (18.1891, -287.1023)
  line L179 (18.1891, -287.1023) -> (18.6734, -284.5341)
  line L180 (18.6734, -284.5341) -> (21.1597, -284.5341)
  line L181 (21.1597, -284.5341) -> (21.1597, -285.1207)
  line L182 (21.1597, -285.1207) -> (19.1645, -285.1207)
  line L183 (19.1645, -285.1207) -> (18.8951, -286.4645)
  spline S679 degree 3 poles (18.8951, -286.4645) (19.0446, -286.373) (19.3354, -286.195) (19.6748, -286.1652) (19.8398, -286.1507) knots 0 0 0 0 0.051785 0.100763 0.100763 0.100763 0.100763
  spline S680 degree 3 poles (19.8398, -286.1507) (20.049, -286.1691) (20.4647, -286.2056) (20.7855, -286.472) (20.9449, -286.6044) knots 0 0 0 0 0.061424 0.122014 0.122014 0.122014 0.122014
  spline S681 degree 3 poles (20.9449, -286.6044) (21.0761, -286.7698) (21.347, -287.1111) (21.3787, -287.5465) (21.3951, -287.7708) knots 0 0 0 0 0.061868 0.12764 0.12764 0.12764 0.12764
  spline S682 degree 3 poles (21.3951, -287.7708) (21.3799, -287.9877) (21.35, -288.4136) (21.1148, -288.7695) (20.9994, -288.9441) knots 0 0 0 0 0.064036 0.125703 0.125703 0.125703 0.125703
  spline S683 degree 3 poles (20.9994, -288.9441) (20.8217, -289.1211) (20.4586, -289.4828) (19.9473, -289.528) (19.6863, -289.5511) knots 0 0 0 0 0.072854 0.148822 0.148822 0.148822 0.148822
  spline S684 degree 3 poles (19.6863, -289.5511) (19.4731, -289.5384) (19.0656, -289.514) (18.7319, -289.2805) (18.5728, -289.1692) knots 0 0 0 0 0.062678 0.119794 0.119794 0.119794 0.119794
  spline S685 degree 3 poles (18.5728, -289.1692) (18.4441, -289.0288) (18.1799, -288.7404) (18.1138, -288.3544) (18.0799, -288.1562) knots 0 0 0 0 0.055877 0.114795 0.114795 0.114795 0.114795
  line L184 (29.5137, -339.4997) -> (29.5136, -335.8776)
  line L185 (29.5136, -335.8776) -> (30.0628, -335.8776)
  line L186 (30.0628, -335.8776) -> (30.0628, -336.3858)
  spline S686 degree 3 poles (30.0628, -336.3858) (30.1247, -336.3012) (30.2495, -336.1307) (30.4269, -336.0157) (30.5164, -335.9577) knots 0 0 0 0 0.031158 0.062835 0.062835 0.062835 0.062835
  spline S687 degree 3 poles (30.5164, -335.9577) (30.6156, -335.9105) (30.8194, -335.8134) (31.0451, -335.8017) (31.161, -335.7957) knots 0 0 0 0 0.032617 0.067048 0.067048 0.067048 0.067048
  spline S688 degree 3 poles (31.161, -335.7957) (31.2855, -335.8004) (31.5179, -335.8093) (31.7249, -335.9141) (31.8209, -335.9628) knots 0 0 0 0 0.036859 0.068796 0.068796 0.068796 0.068796
  spline S689 degree 3 poles (31.8209, -335.9628) (31.9006, -336.0245) (32.0615, -336.1492) (32.143, -336.3358) (32.1842, -336.4301) knots 0 0 0 0 0.029725 0.060035 0.060035 0.060035 0.060035
  spline S690 degree 3 poles (32.1842, -336.4301) (32.3344, -336.2451) (32.6255, -335.8865) (33.0819, -335.8253) (33.3029, -335.7956) knots 0 0 0 0 0.068625 0.133023 0.133023 0.133023 0.133023
  spline S691 degree 3 poles (33.3029, -335.7956) (33.468, -335.8041) (33.7758, -335.8197) (34.0189, -336.0071) (34.1317, -336.0941) knots 0 0 0 0 0.048244 0.08997 0.08997 0.08997 0.08997
  spline S692 degree 3 poles (34.1317, -336.0941) (34.216, -336.2164) (34.4054, -336.4913) (34.4158, -336.8269) (34.4216, -337.0132) knots 0 0 0 0 0.043695 0.098195 0.098195 0.098195 0.098195
  line L187 (34.4216, -337.0132) -> (34.4216, -339.4996)
  line L188 (34.4216, -339.4996) -> (33.8111, -339.4996)
  line L189 (33.8111, -339.4996) -> (33.8111, -337.2179)
  spline S693 degree 3 poles (33.8111, -337.2179) (33.8111, -337.1117) (33.811, -336.9323) (33.7687, -336.7584) (33.7514, -336.6875) knots 0 0 0 0 0.031711 0.053535 0.053535 0.053535 0.053535
  spline S694 degree 3 poles (33.7514, -336.6875) (33.7269, -336.6358) (33.6771, -336.5304) (33.5828, -336.4617) (33.5348, -336.4266) knots 0 0 0 0 0.016863 0.034394 0.034394 0.034394 0.034394
  spline S695 degree 3 poles (33.5348, -336.4266) (33.4791, -336.3978) (33.3636, -336.338) (33.2337, -336.3312) (33.1665, -336.3277) knots 0 0 0 0 0.018597 0.038532 0.038532 0.038532 0.038532
  spline S696 degree 3 poles (33.1665, -336.3277) (33.0453, -336.3375) (32.8074, -336.3568) (32.6227, -336.5077) (32.5321, -336.5818) knots 0 0 0 0 0.035532 0.069798 0.069798 0.069798 0.069798
  spline S697 degree 3 poles (32.5321, -336.5818) (32.4588, -336.6885) (32.2916, -336.9317) (32.284, -337.2286) (32.2797, -337.3953) knots 0 0 0 0 0.038079 0.086792 0.086792 0.086792 0.086792
  line L190 (32.2797, -337.3953) -> (32.2798, -339.4996)
  line L191 (32.2798, -339.4996) -> (31.6659, -339.4996)
  line L192 (31.6659, -339.4996) -> (31.6658, -337.1463)
  spline S698 degree 3 poles (31.6658, -337.1463) (31.6634, -337.0243) (31.6591, -336.8075) (31.5593, -336.616) (31.5157, -336.5324) knots 0 0 0 0 0.036008 0.063954 0.063954 0.063954 0.063954
  spline S699 degree 3 poles (31.5157, -336.5324) (31.4535, -336.4728) (31.3173, -336.3424) (31.1276, -336.3329) (31.0246, -336.3278) knots 0 0 0 0 0.025037 0.054812 0.054812 0.054812 0.054812
  spline S700 degree 3 poles (31.0246, -336.3278) (30.9398, -336.3334) (30.7704, -336.3448) (30.6204, -336.4244) (30.5454, -336.4642) knots 0 0 0 0 0.025173 0.050327 0.050327 0.050327 0.050327
  spline S701 degree 3 poles (30.5454, -336.4642) (30.4768, -336.5159) (30.3364, -336.6215) (30.2637, -336.7815) (30.2265, -336.8633) knots 0 0 0 0 0.025339 0.051812 0.051812 0.051812 0.051812
  spline S702 degree 3 poles (30.2265, -336.8633) (30.1978, -336.9696) (30.131, -337.2171) (30.1288, -337.4739) (30.1276, -337.6204) knots 0 0 0 0 0.032907 0.076633 0.076633 0.076633 0.076633
  line L193 (30.1276, -337.6204) -> (30.1277, -339.4997)
  line L194 (30.1277, -339.4997) -> (29.5137, -339.4997)
  line L195 (18.0812, -338.1903) -> (18.7258, -338.1357)